# Autodesk Inventor part: tube clamp
Saved by Autodesk Inventor 2014 (Build 180170000, 170)
## iProperties
Created: 2016-05-23
Part Number: tube clamp
Material: Generic
Document SubType Name: Modeling
Designer: admin
Density: 1 g/cm^3
Appearance: Default
Author: admin
Autodesk Inventor part; units mm, degrees
ref_plane "YZ Plane" through (0, 0, 0) normal (1, 0, 0) x (0, 1, 0)
ref_plane "XZ Plane" through (0, 0, 0) normal (0, 1, 0) x (-1, 0, 0)
ref_plane "XY Plane" through (0, 0, 0) normal (0, 0, 1) x (1, 0, 0)
ref_plane "Work Plane1" through (0, 0, 0) normal (0, 0, 1) x (1, 0, 0)
ref_plane "Work Plane2" through (0, 0, 0) normal (0, 0, 1) x (1, 0, 0)
sketch "Sketch1" plane through (0, 0, 0) normal (0, 0, 1) x (1, 0, 0)
  circle A0 centre (-0.4764, 18.1938) radius 8.3 projected
  circle A1 centre (-0.4764, 18.1938) radius 6 projected
  circle A2 centre (-0.4764, 18.1938) radius 3.25
  point P0 (0, 0)
  dimension "d0" = 6.5
  constraints: 1 centre point, 1 coincident
  measures "d0" diameter of A2
extrude "Extrusion1" add sketch "Sketch1" along normal blind 6 contours A1
fillet "Fillet1" radius 1 2 edges at (-6.4764, 18.1938, 6) (-6.4764, 18.1938, 0)
ref_plane "Work Plane3" through (-0.4764, 18.1938, 3) normal (0, 0, 1) x (1, 0, 0)
sketch "Sketch2" plane through (-0.4764, 18.1938, 3) normal (0, 0, 1) x (1, 0, 0)
  line L0 (1, 3.4125) -> (-1, 3.4125)
  line L1 (-1, 3.4125) -> (-1, 6.5875)
  line L2 (-1, 6.5875) -> (1, 6.5875)
  line L3 (1, 6.5875) -> (1, 3.4125)
  line L4 (1, 3.4125) -> (-1, 6.5875) construction
  line L5 (-1, 3.4125) -> (1, 6.5875) construction
  circle A0 centre (0, 0) radius 3.25 projected
  point P0 (0.4764, -18.1938)
  point P1 (0, 5)
  dimension "d5" = 2
  dimension "d6" = 5
  constraints: 12 end point, 2 midpoint, 2 parallel, 1 horizontal, 1 perpendicular
  measures "d5" distance between parallel lines of L3 L1
  measures "d6" distance of point (0, 5) A0.centre
extrude "Extrusion2" add sketch "Sketch2" along normal blind 0.5 separate body contours L0 L1 L2 L3
pattern_circular "Circular Pattern1" count 12 over 360 about axis through (-0.4764, 18.1938, 0) along (0, 0, 1) of "Extrusion2" bodies 2
body "Solid1"
body "Solid2"
